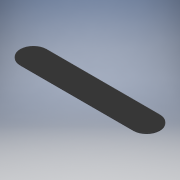
# Autodesk Inventor part: FrontFender
Saved by Autodesk Inventor 2018 (Build 220112000, 112)
## iProperties
Created: 2018-07-29
Part Number: FrontFender
Material: Generic
Document SubType Name: Modeling
Designer: eroldan
Density: 1 g/cm^3
Appearance: Default
Author: eroldan
Autodesk Inventor part; units mm, degrees
ref_plane "YZ Plane" through (0, 0, 0) normal (1, 0, 0) x (0, 1, 0)
ref_plane "XZ Plane" through (0, 0, 0) normal (0, 1, 0) x (-1, 0, 0)
ref_plane "XY Plane" through (0, 0, 0) normal (0, 0, 1) x (1, 0, 0)
sketch "Sketch1" plane through (0, 0, 0) normal (0, 0, 1) x (1, 0, 0)
  line L0 (-215, -50) -> (215, -50)
  line L1 (215, 50) -> (-215, 50)
  arc A0 (215, -50) -> (215, 50) centre (215, 0) ccw
  arc A1 (-215, 50) -> (-215, -50) centre (-215, 0) ccw
  point P0 (0, 0)
  dimension "d2" = 530
  dimension "d3" = 100
  constraints: 4 end point, 4 point on circle, 4 tangent, 2 centre point, 1 horizontal, 1 parallel
  measures "d3" distance between parallel lines of L0 L1
extrude "Extrusion1" add sketch "Sketch1" along normal blind 3
body "Solid1"
